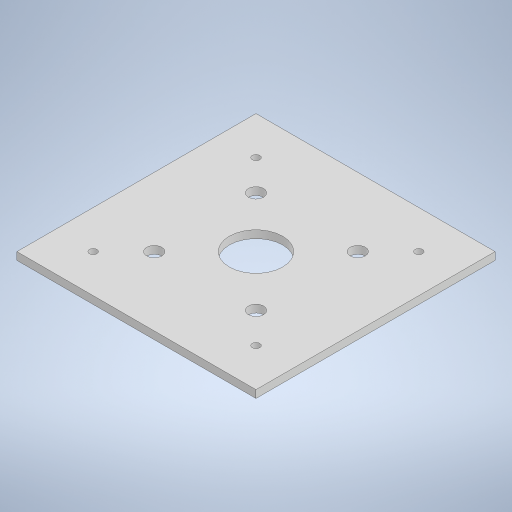
# Autodesk Inventor part: Top Plate
Saved by Autodesk Inventor 2024.1 (Build 281209000, 209)
## iProperties
Created: 2023-12-31
Part Number: Top Plate
Material: Generic
Document SubType Name: Modeling
Designer: ryanm
Density: 1 g/cm^3
Appearance: Default
Author: ryanm
Autodesk Inventor part; units mm, degrees
ref_plane "YZ Plane" through (0, 0, 0) normal (1, 0, 0) x (0, 1, 0)
ref_plane "XZ Plane" through (0, 0, 0) normal (0, 1, 0) x (-1, 0, 0)
ref_plane "XY Plane" through (0, 0, 0) normal (0, 0, 1) x (1, 0, 0)
sketch "Sketch1" plane through (0, 0, 0) normal (0, 1, 0) x (-1, 0, 0)
  line L0 (47, -47) -> (-47, -47)
  line L1 (-47, -47) -> (-47, 47)
  line L2 (-47, 47) -> (47, 47)
  line L3 (47, 47) -> (47, -47)
  point P0 (0, 0)
  point P1 (-47, 0)
  point P2 (0, -47)
  dimension "d0" = 94
  dimension "d1" = 94
  constraints: 8 end point, 2 midpoint, 2 parallel, 1 horizontal, 1 horizontal alignment, 1 perpendicular, 1 vertical alignment
  measures "d0" distance of L1.end L2.end
  measures "d1" distance of L0.end L1.end
extrude "Extrusion1" add sketch "Sketch1" along normal blind 3
sketch "Sketch2" plane through (0, 3, 0) normal (0, 1, 0) x (1, 0, 0)
  line L0 (47, 47) -> (-47, 47) projected
  line L1 (47, -47) -> (47, 47) projected
  line L2 (-47, 47) -> (-47, -47) projected
  line L3 (-47, -47) -> (47, -47) projected
  point P0 (0, 0)
  point P1 (-32, 32)
  point P2 (32, 32)
  point P3 (32, -32)
  point P4 (-32, -32)
  dimension "d4" = 15
  dimension "d5" = 15
  dimension "d6" = 15
  dimension "d7" = 15
  constraints: 2 horizontal alignment, 2 vertical alignment
  measures "d4" distance from line of L0 point (32, 32)
  measures "d5" distance from line of L1 point (32, 32)
  measures "d6" distance from line of L2 point (-32, -32)
  measures "d7" distance from line of L3 point (-32, -32)
hole "Hole1" at (-32, 3, -32) at (32, 3, -32) at (32, 3, 32) at (-32, 3, 32) direction (0, -1, 0) diameter 3 depth 8 tip angle 118
sketch "Sketch3" plane through (0, 3, 0) normal (0, 1, 0) x (1, 0, 0)
  circle A0 centre (0, 0) radius 10.5
  dimension "d15" = 21
  constraints: 1 centre point, 1 coincident
  measures "d15" diameter of A0
extrude "Extrusion2" cut sketch "Sketch3" against normal through all
sketch "Sketch4" plane through (0, 3, 0) normal (0, 1, 0) x (1, 0, 0)
  circle A0 centre (-20, 20) radius 3
  circle A1 centre (20, 20) radius 3
  circle A2 centre (20, -20) radius 3
  circle A3 centre (-20, -20) radius 3
  point P0 (0, 0)
  dimension "d18" = 6
  dimension "d19" = 6
  dimension "d20" = 6
  dimension "d21" = 6
  dimension "d22" = 20
  dimension "d23" = 20
  dimension "d24" = 20
  dimension "d25" = 20
  constraints: 4 centre point, 2 horizontal alignment, 2 vertical alignment
  measures "d18" diameter of A0
  measures "d19" diameter of A1
  measures "d20" diameter of A2
  measures "d21" diameter of A3
  measures "d22" horizontal distance of A1.centre point (0, 0)
  measures "d23" horizontal distance of A0.centre point (0, 0)
  measures "d24" horizontal distance of A0.centre point (0, 0)
  measures "d25" horizontal distance of A3.centre point (0, 0)
extrude "Extrusion3" cut sketch "Sketch4" against normal through all
equation "\"d6\" = d5"
equation "\"d7\" = d4"
equation "\"d23\" = d22"
equation "\"d24\" = d23"
equation "\"d25\" = d24"
body "Solid1"
